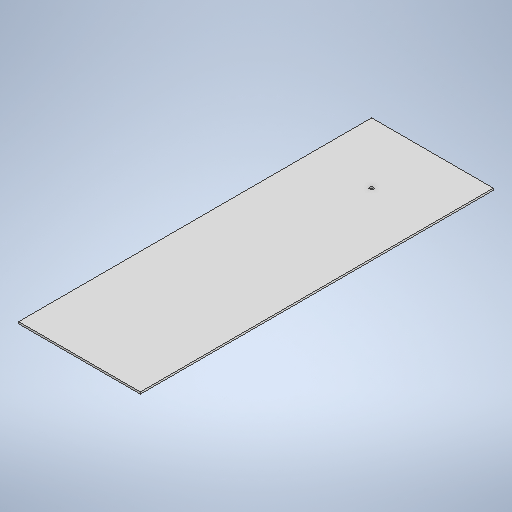
# Autodesk Inventor part: Trebuchet V1 - Long Arm (Sling)
Saved by Autodesk Inventor 2025.2 (Build 292293000, 293)
## iProperties
Created: 2025-04-07
Part Number: Trebuchet V1 - Long Arm (Sling)
Material: Generic
Document SubType Name: Modeling
Designer: Dylan
Density: 1 g/cm^3
Appearance: Default
Author: VRK99-0110
Title: Trebuchet - Long Arm (Sling)
Subject: Trebuchet Project
Autodesk Inventor part; units mm, degrees
ref_plane "YZ Plane" through (0, 0, 0) normal (1, 0, 0) x (0, 1, 0)
ref_plane "XZ Plane" through (0, 0, 0) normal (0, 1, 0) x (-1, 0, 0)
ref_plane "XY Plane" through (0, 0, 0) normal (0, 0, 1) x (1, 0, 0)
sketch "Sketch1" plane through (0, 0, 0) normal (0, 1, 0) x (-1, 0, 0)
  line L0 (0, 0) -> (200, 0)
  line L1 (200, 0) -> (200, -480)
  line L2 (200, -480) -> (0, -480)
  line L3 (0, -480) -> (0, 0)
  line L4 (0, -480) -> (100, -480)
  line L5 (200, -480) -> (200, -580)
  line L6 (200, -580) -> (0, -580)
  line L7 (0, -580) -> (0, -480)
  dimension "d0" = 200
  dimension "d1" = 480
  constraints: 16 end point, 5 perpendicular, 1 horizontal, 1 midpoint, 1 vertical
  measures "d0" distance of L0.start L0.end
  measures "d1" distance of L0.end L1.end
extrude "Extrusion1" add sketch "Sketch1" along normal blind 3.175
sketch "Sketch2" plane through (0, 3.175, 0) normal (0, 1, 0) x (1, 0, 0)
  circle A0 centre (-100, 480) radius 3.175
  point P0 (0, 0)
  dimension "d5" = 6.35
  constraints: 1 centre point
  measures "d5" diameter of A0
extrude "Extrusion2" cut sketch "Sketch2" against normal blind 3.175
body "Solid1"
